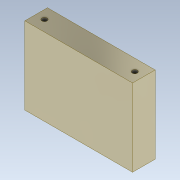
# Autodesk Inventor part: base_soportes
Saved by Autodesk Inventor 2022 (Build 260153000, 153)
## iProperties
Created: 2022-11-16
Part Number: base_soportes
Material: Generic
Document SubType Name: Modeling
Designer: ferna
Density: 1 g/cm^3
Appearance: Nickel
Author: ferna
Autodesk Inventor part; units mm, degrees
ref_plane "YZ Plane" through (0, 0, 0) normal (1, 0, 0) x (0, 1, 0)
ref_plane "XZ Plane" through (0, 0, 0) normal (0, 1, 0) x (-1, 0, 0)
ref_plane "XY Plane" through (0, 0, 0) normal (0, 0, 1) x (1, 0, 0)
sketch "Sketch1" plane through (0, 0, 0) normal (0, 1, 0) x (-1, 0, 0)
  line L0 (0, 0) -> (124, 0)
  line L1 (124, 0) -> (124, -26)
  line L2 (124, -26) -> (0, -26)
  line L3 (0, -26) -> (0, 0)
  circle A0 centre (10.0002, -12.5957) radius 3
  circle A1 centre (114, -12.5957) radius 3
  line L4 (0, 0) -> (124.0002, 0)
  line L5 (124.0002, 0) -> (124.0002, -2.5957)
  line L6 (124.0002, -2.5957) -> (117, -2.5957)
  line L7 (117, -2.5957) -> (117, -5.5957)
  line L8 (117, -5.5957) -> (124.0002, -5.5957)
  line L9 (124.0002, -5.5957) -> (124.0002, -19.5957)
  line L10 (124.0002, -19.5957) -> (117, -19.5957)
  line L11 (117, -19.5957) -> (117, -22.5957)
  line L12 (117, -22.5957) -> (124.0002, -22.5957)
  line L13 (124.0002, -22.5957) -> (124.0002, -26)
  line L14 (124.0002, -26) -> (0, -26)
  line L15 (0, -26) -> (0, -22.5957)
  line L16 (0, -22.5957) -> (7, -22.5957)
  line L17 (7, -22.5957) -> (7, -19.5957)
  line L18 (7, -19.5957) -> (0, -19.5957)
  line L19 (0, -19.5957) -> (0, -5.5957)
  line L20 (0, -5.5957) -> (7, -5.5957)
  line L21 (7, -5.5957) -> (7, -2.5957)
  line L22 (7, -2.5957) -> (0, -2.5957)
  line L23 (0, -2.5957) -> (0, 0)
  line L24 (31.0002, -9.0957) -> (28.0002, -9.0957)
  line L25 (28.0002, -9.0957) -> (28.0002, -16.0957)
  line L26 (28.0002, -16.0957) -> (31.0002, -16.0957)
  line L27 (31.0002, -16.0957) -> (31.0002, -9.0957)
  line L28 (31.0002, -5.5957) -> (22, -5.5957)
  line L29 (22, -5.5957) -> (22, -2.5957)
  line L30 (22, -2.5957) -> (54.5, -2.5957)
  line L31 (54.5, -2.5957) -> (54.5, -5.5957)
  line L32 (54.5, -5.5957) -> (31.0002, -5.5957)
  line L33 (28.0002, -19.5957) -> (54.5, -19.5957)
  line L34 (54.5, -19.5957) -> (54.5, -22.5957)
  line L35 (54.5, -22.5957) -> (22, -22.5957)
  line L36 (22, -22.5957) -> (22, -19.5957)
  line L37 (22, -19.5957) -> (28.0002, -19.5957)
  line L38 (69.5, -5.5957) -> (69.5, -2.5957)
  line L39 (69.5, -2.5957) -> (102, -2.5957)
  line L40 (102, -2.5957) -> (102, -5.5957)
  line L41 (102, -5.5957) -> (69.5, -5.5957)
  line L42 (93, -9.0957) -> (96, -9.0957)
  line L43 (96, -9.0957) -> (96, -16.0957)
  line L44 (96, -16.0957) -> (93, -16.0957)
  line L45 (93, -16.0957) -> (93, -9.0957)
  line L46 (96, -19.5957) -> (69.5, -19.5957)
  line L47 (69.5, -19.5957) -> (69.5, -22.5957)
  line L48 (69.5, -22.5957) -> (102, -22.5957)
  line L49 (102, -22.5957) -> (102, -19.5957)
  line L50 (102, -19.5957) -> (96, -19.5957)
  dimension "d0" = 124
  dimension "d1" = 26
  dimension "d4" = 124.0002
  dimension "d5" = 26
  constraints: 102 end point, 2 centre point, 2 parallel, 1 horizontal, 1 perpendicular
  measures "d0" distance of L1.end L2.end
  measures "d1" distance of L0.end L1.end
  measures "d4" distance between parallel lines of L3 L9
  measures "d5" distance between parallel lines of L0 L14
extrude "Extrusion1" add sketch "Sketch1" along normal blind 89 contours L0 L1 L6 L7 L8 L10 L11 L12 L2 L3 L16 L17 L18 L20 L21 L22 | L22 L21 L20 L3 | L1 L8 L7 L6 | L18 L17 L16 L3 | L1 L12 L11 L10 | A0 | A1 | L27 L26 L25 L24 | L28 L29 L30 L31 L32 | L33 L34 L35 L36 L37 | L38 L39 L40 L41 | L42 L43 L44 L45 | L50 L49 L48 L47 L46
sketch "Sketch2" plane through (0, 89, 0) normal (0, 1, 0) x (1, 0, 0)
  line L0 (0, 0) -> (-124, 0)
  line L1 (-124, 0) -> (-124, 26)
  line L2 (-124, 26) -> (0, 26)
  line L3 (0, 26) -> (0, 0)
  line L4 (-28.0002, 16.0957) -> (-31.0002, 16.0957)
  line L5 (-31.0002, 16.0957) -> (-31.0002, 9.0957)
  line L6 (-31.0002, 9.0957) -> (-28.0002, 9.0957)
  line L7 (-31.0002, 5.5957) -> (-22, 5.5957)
  circle A0 centre (-10.0002, 12.5957) radius 3
  line L8 (-54.5, 2.5957) -> (-54.5, 5.5957)
  line L9 (-22, 2.5957) -> (-54.5, 2.5957)
  line L10 (-69.5, 5.5957) -> (-69.5, 2.5957)
  circle A1 centre (-114, 12.5957) radius 3
  line L11 (0, 0) -> (-124.0002, 0)
  line L12 (-124.0002, 26) -> (0, 26)
  line L13 (-117, 5.5957) -> (-124.0002, 5.5957)
  line L14 (-117, 19.5957) -> (-117, 22.5957)
  line L15 (-124.0002, 5.5957) -> (-124.0002, 19.5957)
  line L16 (-124.0002, 19.5957) -> (-117, 19.5957)
  line L17 (-117, 2.5957) -> (-117, 5.5957)
  line L18 (-124.0002, 2.5957) -> (-117, 2.5957)
  line L19 (-124.0002, 0) -> (-124.0002, 2.5957)
  line L20 (-124.0002, 22.5957) -> (-124.0002, 26)
  line L21 (-117, 22.5957) -> (-124.0002, 22.5957)
  line L22 (-102, 19.5957) -> (-96, 19.5957)
  line L23 (-102, 22.5957) -> (-102, 19.5957)
  line L24 (-96, 16.0957) -> (-93, 16.0957)
  line L25 (-93, 16.0957) -> (-93, 9.0957)
  line L26 (-93, 9.0957) -> (-96, 9.0957)
  line L27 (-96, 9.0957) -> (-96, 16.0957)
  line L28 (-96, 19.5957) -> (-69.5, 19.5957)
  line L29 (-69.5, 2.5957) -> (-102, 2.5957)
  line L30 (-102, 2.5957) -> (-102, 5.5957)
  line L31 (-102, 5.5957) -> (-69.5, 5.5957)
  line L32 (-69.5, 22.5957) -> (-102, 22.5957)
  line L33 (-69.5, 19.5957) -> (-69.5, 22.5957)
  line L34 (-54.5, 5.5957) -> (-31.0002, 5.5957)
  line L35 (-28.0002, 9.0957) -> (-28.0002, 16.0957)
  line L36 (-54.5, 22.5957) -> (-22, 22.5957)
  line L37 (-28.0002, 19.5957) -> (-54.5, 19.5957)
  line L38 (-54.5, 19.5957) -> (-54.5, 22.5957)
  line L39 (-22, 19.5957) -> (-28.0002, 19.5957)
  line L40 (-22, 22.5957) -> (-22, 19.5957)
  line L41 (-22, 5.5957) -> (-22, 2.5957)
  line L42 (0, 26) -> (0, 22.5957)
  line L43 (0, 22.5957) -> (-7, 22.5957)
  line L44 (-7, 22.5957) -> (-7, 19.5957)
  line L45 (-7, 19.5957) -> (0, 19.5957)
  line L46 (0, 19.5957) -> (0, 5.5957)
  line L47 (0, 5.5957) -> (-7, 5.5957)
  line L48 (-7, 2.5957) -> (0, 2.5957)
  line L49 (0, 2.5957) -> (0, 0)
  line L50 (-7, 5.5957) -> (-7, 2.5957)
  dimension "d6" = 124
  dimension "d7" = 26
  dimension "d8" = 124.0002
  dimension "d9" = 26
  constraints: 102 end point, 2 centre point, 2 parallel, 1 perpendicular
  measures "d6" distance of L1.end L2.end
  measures "d7" distance of L0.end L1.end
  measures "d8" distance between parallel lines of L3 L15
  measures "d9" distance between parallel lines of L0 L12
extrude "Extrusion2" cut sketch "Sketch2" against normal blind 10 contours A0 | A1
thread "Thread1" size "M6x1" class "6H" standard "ANSI Metric M Profile" full length
thread "Thread2" size "M6x1" class "6H" standard "ANSI Metric M Profile" full length
body "Solid1"
